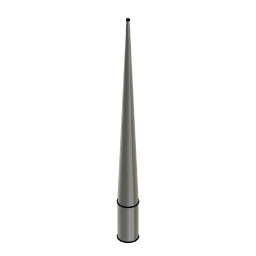
assembly_linear_actuator_no_spring (Autodesk Fusion 360 archive; units mm, degrees)
design "single tip press fit"
Autodesk Fusion 360 part; units mm, degrees
sketch "Sketch1" plane through (0, 0, 0) normal (0, 0, 1) x (1, 0, 0)
  circle A0 centre (0, 0) radius 1.5875
  dimension "d1" = 3.175
  dimension "d6" = 0
  constraint coincident A0.centre origin
  measures "d1" diameter of A0
ref_plane "WorkPlane1" through (0, 0, 33.02) normal (0, 0, 1) x (1, 0, 0)
sketch "Sketch2" plane through (0, 0, 33.02) normal (0, 0, 1) x (1, 0, 0)
  circle A0 centre (0, 0) radius 0.254
  dimension "d3" = 0.508
  constraint coincident A0.centre origin
  measures "d3" diameter of A0
loft "Loft1" add profiles "Sketch1", "Sketch2" section 1 section 2
extrude "Extrude2" add 1 faces at (-0.3879, 0.3599, 0) along direction (0, 0, -1) blind 6.35
sketch "Sketch4" plane through (0, 0, 0) normal (0, 1, 0) x (1, 0, 0)
equation "d1 = ( 1 / 8 ) * 1 in"

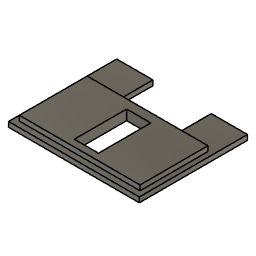
design "table_window"
Autodesk Fusion 360 part; units mm, degrees
sketch "Sketch1" plane through (0, 0, 0) normal (0, 0, 1) x (1, 0, 0)
  line L0 (0, 0) -> (76.2, 0)
  line L1 (76.2, 0) -> (76.2, 42.8752)
  line L2 (76.2, 42.8752) -> (0, 42.8752)
  line L3 (0, 42.8752) -> (0, 0)
  line L4 (38.1, 42.8752) -> (38.1, 0) construction
  line L5 (0, 21.4376) -> (76.2, 20.5486) construction
  line L6 (30.48, 4.2545) -> (45.72, 4.2545)
  line L7 (79.375, -3.6195) -> (-3.175, -3.6195)
  line L8 (-3.175, -3.6195) -> (-3.175, 45.6057)
  line L9 (-3.175, 45.6057) -> (79.375, 45.6057)
  line L10 (79.375, 45.6057) -> (79.375, -3.6195)
  line L11 (74.796, 42.8752) -> (79.375, 45.6057) construction
  line L12 (-3.175, -3.6195) -> (2.8949, 0) construction
  line L13 (79.375, -3.6195) -> (73.3051, 0) construction
  line L14 (1.404, 42.8752) -> (-3.175, 45.6057) construction
  line L15 (45.72, 37.2745) -> (30.48, 37.2745)
  line L16 (45.72, 37.2745) -> (45.72, 4.2545)
  line L17 (30.48, 37.2745) -> (30.48, 4.2545)
  dimension "d1" = 76.2
  dimension "d2" = 42.8752
  dimension "d3" = 15.24
  dimension "d5" = 82.55
  dimension "d6" = 49.2252
  constraint horizontal L0
  constraint vertical L1
  constraint horizontal L2
  constraint vertical L3
  constraint coincident L0.start L3.end
  constraint midpoint L2 L4.start
  constraint midpoint L0 L4.end
  constraint midpoint L3 L5.start
  constraint coincident L1 L5.end
  constraint horizontal L7
  constraint perpendicular L7 L8
  constraint parallel L7 L9
  constraint parallel L8 L10
  constraint coincident L2 L11.start
  constraint collinear L11 L12
  constraint coincident L0 L12.end
  constraint coincident L0 L13.end
  constraint collinear L13 L14
  constraint coincident L2 L14.start
  constraint horizontal L15
  constraint perpendicular L6 L17
  measures "d1" distance of L0.start L0.end
  measures "d2" distance of L0.start L2.end
  measures "d3" distance of L6.start L6.end
  measures "d5" distance of L8.end L9.end
  measures "d6" distance of L7.end L8.end
extrude "Extrude1" add sketch "Sketch1" along normal blind 6.35 contours L0 L1 L2 L3
extrude "Extrude2" add sketch "Sketch1" along normal blind 3.175 contours L7 L8 L9 L10
sketch "Sketch2" plane through (0, 45.6057, 0) normal (0, 1, 0) x (-1, 0, 0)
  line L0 (-79.375, 0) -> (3.175, 0)
  line L1 (3.175, 0) -> (3.175, 3.175)
  line L2 (3.175, 3.175) -> (-79.375, 3.175)
  line L3 (-79.375, 3.175) -> (-79.375, 0)
  line L4 (3.175, 0) -> (-19.685, 0)
  line L5 (-19.685, 0) -> (-19.685, 3.175)
  line L6 (-19.685, 3.175) -> (3.175, 3.175)
  line L7 (3.175, 3.175) -> (3.175, 0)
  line L8 (-79.375, 0) -> (-56.515, 0)
  line L9 (-56.515, 0) -> (-56.515, 3.175)
  line L10 (-56.515, 3.175) -> (-79.375, 3.175)
  line L11 (-79.375, 3.175) -> (-79.375, 0)
  dimension "d12" = 22.86
  dimension "d13" = 22.86
  constraint horizontal L4
  constraint vertical L5
  constraint horizontal L6
  constraint vertical L7
  constraint coincident L0.end L1.start
  constraint horizontal L8
  constraint vertical L9
  constraint horizontal L10
  constraint vertical L11
  constraint coincident L0.start L3.end
  measures "d12" distance of L0.end L4.end
  measures "d13" distance of L0.start L8.end
extrude "Extrude3" add sketch "Sketch2" along normal blind 19.05 contours L0 L2 L3 L8 L9 L10 L11 | L0 L1 L2 L4 L5 L6 L7

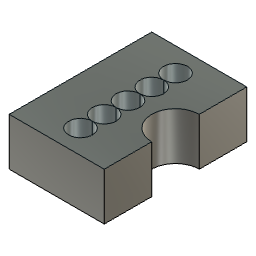
design "base for 5 tips press fit"
Autodesk Fusion 360 part; units mm, degrees
sketch "Sketch1" plane through (0, 0, 0) normal (0, 0, 1) x (1, 0, 0)
  line L0 (-6.35, 9.525) -> (6.35, 9.525)
  line L1 (6.35, 9.525) -> (6.35, -9.525)
  line L2 (6.35, -9.525) -> (-6.35, -9.525)
  line L3 (-6.35, -9.525) -> (-6.35, 9.525)
  line L4 (0, 0) -> (0, 3.175) construction
  line L5 (0, 3.175) -> (0, 6.35) construction
  line L6 (0, 0) -> (0, -3.175) construction
  line L7 (0, -3.175) -> (0, -6.35) construction
  circle A0 centre (0, 6.35) radius 1.5875
  circle A1 centre (0, 3.175) radius 1.5875
  circle A2 centre (0, 0) radius 1.5875
  circle A3 centre (0, -3.175) radius 1.5875
  circle A4 centre (0, -6.35) radius 1.5875
  arc A5 (6.35, 3.175) -> (6.35, -3.175) centre (6.35, 0) ccw
  dimension "d3" = 12.7
  dimension "d4" = 19.05
  dimension "d5" = 3.175
  dimension "d6" = 3.175
  dimension "d7" = 3.175
  dimension "d8" = 3.175
  dimension "d9" = 3.175
  dimension "d10" = 3.175
  dimension "d11" = 3.175
  dimension "d12" = 3.175
  dimension "d13" = 3.175
  dimension "d21" = 6.35
  constraint horizontal L0
  constraint vertical L1
  constraint horizontal L2
  constraint vertical L3
  constraint coincident L4.start L6.start
  constraint vertical L4
  constraint parallel L4 L5
  constraint parallel L4 L6
  constraint parallel L6 L7
  constraint coincident L5.end A0.centre
  constraint coincident L4.end L5.start
  constraint coincident L6.end L7.start
  constraint coincident L7.end A4.centre
  constraint midpoint L1 A5.centre
  constraint coincident L1 A5.end
  constraint coincident L1 A5.start
  measures "d3" distance of L0.start L0.end
  measures "d4" distance of L0.start L2.end
  measures "d5" distance of L4.start L4.end
  measures "d6" distance of L4.end L5.end
  measures "d7" distance of L4.start L6.end
  measures "d8" distance of L6.end L7.end
  measures "d9" diameter of A0
  measures "d10" diameter of A1
  measures "d11" diameter of A2
  measures "d12" diameter of A3
  measures "d13" diameter of A4
  measures "d21" diameter of A5
extrude "Extrude1" add sketch "Sketch1" along normal blind 6.35 contours L0 L1 L2 L3 A5
sketch "Sketch2" plane through (0, 0, 6.35) normal (0, 0, 1) x (-1, 0, 0)
  circle A0 centre (0, 6.35) radius 1.5875
  circle A1 centre (0, -6.35) radius 1.5875
  line L0 (6.35, 9.525) -> (-6.35, 9.525)
  line L1 (-6.35, -3.175) -> (-6.35, -9.525)
  line L2 (-6.35, -9.525) -> (6.35, -9.525)
  line L3 (6.35, -9.525) -> (6.35, 9.525)
  arc A2 (1.905, 6.35) -> (-1.905, 6.35) centre (0, 6.35) ccw
  arc A3 (-1.905, -6.35) -> (1.905, -6.35) centre (0, -6.35) ccw
  circle A4 centre (0, -3.175) radius 1.5875
  arc A5 (0, -1.5875) -> (0, 1.5875) centre (0, 0) ccw
  arc A6 (0, 1.5875) -> (0, 4.7625) centre (0, 3.175) ccw
  arc A7 (0, -1.5875) -> (0, -4.7625) centre (0, -3.175) ccw
  arc A8 (0, 1.5875) -> (0, -1.5875) centre (0, 0) ccw
  arc A9 (0, 4.7625) -> (0, 1.5875) centre (0, 3.175) ccw
  line L4 (-6.35, 9.525) -> (-6.35, 3.175)
  arc A10 (-6.35, -3.175) -> (-6.35, 3.175) centre (-6.35, 0) ccw
  dimension "d17" = 3.81
  dimension "d18" = 3.81
  constraint concentric A0 A2
  constraint coincident L3 A2.start
  constraint concentric A1 A3
  measures "d17" diameter of A2
  measures "d18" diameter of A3
sketch "Sketch3" plane through (0, 0, 6.35) normal (0, 0, 1) x (-1, 0, 0)
  circle A0 centre (0, 6.35) radius 1.5875
  arc A1 (0, 1.5875) -> (0, 4.7625) centre (0, 3.175) ccw
  arc A2 (0, -1.5875) -> (0, 1.5875) centre (0, 0) ccw
  arc A3 (0, -4.7625) -> (0, -1.5875) centre (0, -3.175) ccw
  circle A4 centre (0, -6.35) radius 1.5875
  arc A5 (0, -1.5875) -> (0, -4.7625) centre (0, -3.175) ccw
  arc A6 (0, 1.5875) -> (0, -1.5875) centre (0, 0) ccw
  arc A7 (0, 4.7625) -> (0, 1.5875) centre (0, 3.175) ccw
  line L0 (-6.35, -3.175) -> (-6.35, -9.525)
  line L1 (-6.35, -9.525) -> (6.35, -9.525)
  line L2 (6.35, -9.525) -> (6.35, 9.525)
  line L3 (6.35, 9.525) -> (-6.35, 9.525)
  line L4 (-6.35, 9.525) -> (-6.35, 3.175)
  arc A8 (-6.35, -3.175) -> (-6.35, 3.175) centre (-6.35, 0) ccw
sketch "Sketch4" plane through (-6.35, 0, 0) normal (-1, 0, 0) x (0, -1, 0)
  line L0 (-9.525, 0) -> (9.525, 0)
  line L1 (9.525, 0) -> (9.525, 6.35)
  line L2 (9.525, 6.35) -> (-9.525, 6.35)
  line L3 (-9.525, 6.35) -> (-9.525, 0)
  line L4 (0, 0) -> (0, 3.175) construction
  circle A0 centre (0, 3.175) radius 1.905
  dimension "d22" = 3.175
  dimension "d23" = 3.81
  constraint coincident L4.start origin
  constraint perpendicular L0 L4
  constraint coincident L4.end A0.centre
  measures "d22" distance of L4.start L4.end
  measures "d23" diameter of A0
extrude "Extrude3" cut sketch "Sketch4" against normal blind 3.81 contours A0
thread "Thread1" "ANSI Unified Screw Threads 0.164(#8) 8-32 UNC 3B" major diameter 4.1656 minor diameter 3.4163 pitch 0.7937 angle 60 resizes the face on face at (-3.81, -1.8955, 2.9853)
equation "d9 = ( 1 / 8 ) * 1 in"
equation "d10 = ( 1 / 8 ) * 1 in"
equation "d11 = ( 1 / 8 ) * 1 in"
equation "d13 = ( 1 / 8 ) * 1 in"
equation "d21 = ( 1 / 4 ) * 1 in"
equation "d22 = ( 1 / 8 ) * 1 in"

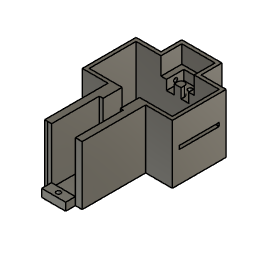
design "Circuit Base new"
Autodesk Fusion 360 part; units mm, degrees
sketch "Sketch1" plane through (0, 0, 0) normal (0, 0, 1) x (1, 0, 0)
  line L0 (76.2, 25.4) -> (0, 25.4)
  line L1 (48.6484, -35) -> (48.6484, -85)
  line L2 (26.6484, -76) -> (26.6484, -85)
  line L3 (48.6484, -76) -> (48.6484, -35)
  line L4 (26.6484, -35) -> (26.6484, -76)
  line L5 (30.1, -17.526) -> (30.1, -34.9936)
  line L6 (46.1, -34.9936) -> (46.1, -17.526)
  circle A0 centre (37.6484, -83.3194) radius 2.05
  line L7 (37.6484, -81.2694) -> (37.6484, -80.5) construction
  line L8 (48.6484, -76.0942) -> (48.6484, -35)
  line L9 (26.6484, -75.9063) -> (26.6484, -35)
  line L10 (46.1, -17.526) -> (46.1, -34.9936)
  line L11 (30.1, -34.9936) -> (26.6484, -34.9936)
  line L12 (30.1, -17.526) -> (30.1, -34.9936)
  line L13 (0, 25.4) -> (76.2, 25.4)
  line L14 (79.375, 28.575) -> (-3.175, 28.575)
  line L15 (30.1, -17.526) -> (30.1, -34.9936)
  line L16 (30.1, -34.9936) -> (26.6484, -34.9936)
  line L17 (26.6484, -34.9936) -> (26.6484, -75.9063)
  line L18 (46.1, -17.526) -> (46.1, -34.9936)
  line L19 (46.1, -34.9936) -> (48.6484, -34.9936)
  line L20 (48.6484, -34.9936) -> (48.6484, -76.0942)
  line L21 (46.1, -34.9936) -> (48.6484, -34.9936)
  line L22 (26.6484, -75.9063) -> (26.6484, -78.7257)
  line L23 (26.6484, -78.7257) -> (48.6484, -78.9136)
  line L24 (48.6484, -85) -> (48.6484, -78.9136)
  line L25 (48.6484, -76.0942) -> (48.6484, -76)
  line L26 (26.6484, -85) -> (26.6484, -78.7257)
  line L27 (26.6484, -75.9063) -> (26.6484, -35)
  line L28 (52.3234, -78.9136) -> (48.6484, -78.9136)
  line L29 (22.9734, -78.7257) -> (26.6484, -78.7257)
  line L30 (26.6484, -85) -> (26.6484, -87.8194)
  line L31 (48.6484, -85) -> (48.6484, -87.8194)
  line L32 (48.6484, -87.8194) -> (26.6484, -87.8194)
  line L33 (20.32, -78.74) -> (20.32, -66.04)
  line L34 (20.32, -66.04) -> (20.32, -20.701)
  line L35 (22.9734, -78.7257) -> (20.32, -78.74)
  line L36 (52.3234, -78.9136) -> (54.8634, -78.9136)
  line L37 (54.8634, -78.9136) -> (54.8634, -20.701)
  line L38 (-3.1761, -11.938) -> (-3.175, -11.938)
  line L39 (76.1981, -17.526) -> (46.1, -17.526)
  line L40 (30.1, -17.526) -> (0, -17.526)
  line L41 (-3.173, -20.701) -> (20.32, -20.701)
  line L42 (54.8634, -20.701) -> (79.3731, -20.701)
  line L43 (76.2, 25.4) -> (76.1981, -17.526)
  line L44 (79.375, 28.575) -> (79.3731, -20.701)
  line L45 (0, 25.4) -> (0, -17.526)
  line L46 (-3.175, 28.575) -> (-3.173, -20.701)
  point P0 (38.1, 0)
  point P1 (38.1, -15)
  point P2 (37.6484, 0)
  dimension "d2" = 25.4
  dimension "d5" = 9
  dimension "d6" = 41
  dimension "d9" = 16
  dimension "d12" = 4.1
  dimension "d47" = 2.8194
  dimension "d48" = 2.8194
  dimension "d50" = 2.8194
  dimension "d51" = 2.8194
  dimension "d53" = 2.54
  constraint horizontal L0
  constraint vertical L1
  constraint vertical L26
  constraint vertical L24
  constraint vertical L2
  constraint vertical L3
  constraint vertical L4
  constraint parallel L5 L6
  constraint vertical L8
  constraint vertical L9
  constraint horizontal L21
  constraint vertical L10
  constraint horizontal L11
  constraint vertical L12
  constraint horizontal L13
  constraint horizontal L14
  constraint vertical L15
  constraint horizontal L16
  constraint vertical L17
  constraint vertical L18
  constraint horizontal L19
  constraint vertical L20
  constraint collinear L24 L25
  constraint collinear L26 L27
  constraint coincident A0 L7.start
  constraint perpendicular L29 L33
  constraint coincident L5.start L39
  constraint collinear L39 L40
  constraint collinear L41 L42
  constraint vertical L45
  measures "d2" distance of origin L0.end
  measures "d5" distance of L2.end L2.start
  measures "d6" distance of L2.start L4.start
  measures "d9" distance of L5.end L6.start
  measures "d12" diameter of A0
  measures "d47" distance of L9.start L22.end
  measures "d48" distance of L8.start L23.end
  measures "d50" distance of L2.end L30.end
  measures "d51" distance of L1.end L31.end
  measures "d53" distance of L28.start L36.end
extrude "Extrude7" add sketch "Sketch1" against normal blind 3.175 makes body 1
extrude "Extrude8" add sketch "Sketch1" along normal blind 50.8 contours L0 L1 L2 L3 L4 L5 L6 L8 L9 L10 L11 L12 L13 L14 L15 L16 L17 L18 L19 L20 L21 L22 L25 L27 L28 L29 L33 L34 L35 L36 L37 L39 L40 L41 L42 L43 L44 L45 L46 bodies 1
extrude "Extrude10" add sketch "Sketch1" along normal blind 4 contours L1 L2 L23 L24 L26 L30 L31 L32 bodies 1
sketch "Sketch3" plane through (0, 28.575, 0) normal (0, 1, 0) x (-1, 0, 0)
  line L0 (-79.375, 50.8) -> (-79.375, -3.175)
  line L1 (-79.375, -3.175) -> (3.175, -3.175)
  line L2 (3.175, -3.175) -> (3.175, 50.8)
  line L3 (3.175, 50.8) -> (-79.375, 50.8)
  line L4 (-53.34, 20.32) -> (-22.86, 20.32)
  line L5 (-22.86, 20.32) -> (-22.86, 34.6202)
  line L6 (-22.86, 34.6202) -> (-53.34, 34.6202)
  line L7 (-53.34, 34.6202) -> (-53.34, 20.32)
  dimension "d87" = 30.48
  dimension "d88" = 14.3002
  constraint horizontal L4
  constraint vertical L5
  constraint horizontal L6
  constraint vertical L7
  measures "d87" distance of L4.start L4.end
  measures "d88" distance of L4.start L6.end
extrude "Extrude11" add sketch "Sketch3" along normal blind 15.875 separate body contours L4 L5 L6 L7 makes body 2
sketch "Sketch4" plane through (0, 0, 34.6202) normal (0, 0, 1) x (-1, 0, 0)
  line L0 (-22.86, -28.575) -> (-53.34, -28.575)
  line L1 (-53.34, -28.575) -> (-53.34, -44.45)
  line L2 (-53.34, -44.45) -> (-22.86, -44.45)
  line L3 (-22.86, -44.45) -> (-22.86, -28.575)
  line L4 (-48.26, -28.575) -> (-27.94, -28.575)
  line L5 (-27.94, -28.575) -> (-27.94, -41.275)
  line L6 (-27.94, -41.275) -> (-48.26, -41.275)
  line L7 (-48.26, -41.275) -> (-48.26, -28.575)
  circle A0 centre (-38.1, -28.575) radius 3.175
  dimension "d91" = 20.32
  dimension "d92" = 12.7
  dimension "d93" = 5.08
  dimension "d94" = 6.35
  constraint horizontal L4
  constraint vertical L5
  constraint horizontal L6
  constraint vertical L7
  constraint coincident L0 L4.start
  constraint midpoint L4 A0.centre
  measures "d91" distance of L4.start L4.end
  measures "d92" distance of L4.start L6.end
  measures "d93" distance of L3 L5
  measures "d94" diameter of A0
extrude "Extrude12" cut sketch "Sketch4" against normal blind 8.89 contours L0 L4 L5 L6 L7 A0 bodies 2
sketch "Sketch5" plane through (22.86, 0, 0) normal (-1, 0, 0) x (0, -1, 0)
  line L0 (-28.575, 20.32) -> (-28.575, 34.6202)
  line L1 (-28.575, 34.6202) -> (-44.45, 34.6202)
  line L2 (-44.45, 34.6202) -> (-44.45, 20.32)
  line L3 (-44.45, 20.32) -> (-28.575, 20.32)
  circle A0 centre (-33.7311, 29.984) radius 1.778
  dimension "d97" = 3.556
  measures "d97" diameter of A0
extrude "Extrude13" cut sketch "Sketch5" against normal blind 48.26 contours A0 bodies 2
extrude "Extrude14" add 1 faces at (43.18, 44.45, 25.0867) along direction (0, 1, 0) blind 3.175 on bodies 2 bodies 2
extrude "Extrude15" add 1 faces at (22.86, 43.56, 28.1334) along direction (-1, 0, 0) blind 3.175 on bodies 2 bodies 1 2
extrude "Extrude16" add 1 faces at (53.34, 43.56, 28.1334) along direction (1, 0, 0) blind 3.175 on bodies 1 bodies 1
extrude "Extrude17" add 1 faces at (22.4367, 39.1583, 34.6202) along direction (0, 0, 1) up to surface (16.1798 mm away) on bodies 1 bodies 1
sketch "Sketch6" plane through (0, 0, 50.8) normal (0, 0, 1) x (-1, 0, 0)
  line L0 (-48.26, -28.575) -> (-27.94, -28.575)
  line L1 (-27.94, -28.575) -> (-27.94, -41.275)
  line L2 (-27.94, -41.275) -> (-48.26, -41.275)
  line L3 (-48.26, -41.275) -> (-48.26, -28.575)
  line L4 (-56.515, -28.575) -> (-56.515, -47.625)
  line L5 (-56.515, -47.625) -> (-19.685, -47.625)
  line L6 (-19.685, -47.625) -> (-19.685, -28.575)
  line L7 (-19.685, -28.575) -> (3.175, -28.575)
  line L8 (3.175, -28.575) -> (3.173, 20.701)
  line L9 (3.173, 20.701) -> (-20.32, 20.701)
  line L10 (-20.32, 20.701) -> (-20.32, 78.74)
  line L11 (-20.32, 78.74) -> (-22.9734, 78.7257)
  line L12 (-22.9734, 78.7257) -> (-26.6484, 78.7257)
  line L13 (-26.6484, 78.7257) -> (-26.6484, 34.9936)
  line L14 (-26.6484, 34.9936) -> (-30.1, 34.9936)
  line L15 (-30.1, 34.9936) -> (-30.1, 17.526)
  line L16 (-30.1, 17.526) -> (0, 17.526)
  line L17 (0, 17.526) -> (0, -25.4)
  line L18 (0, -25.4) -> (-76.2, -25.4)
  line L19 (-76.2, -25.4) -> (-76.1981, 17.526)
  line L20 (-76.1981, 17.526) -> (-46.1, 17.526)
  line L21 (-46.1, 17.526) -> (-46.1, 34.9936)
  line L22 (-46.1, 34.9936) -> (-48.6484, 34.9936)
  line L23 (-48.6484, 34.9936) -> (-48.6484, 78.9136)
  line L24 (-48.6484, 78.9136) -> (-54.8634, 78.9136)
  line L25 (-54.8634, 78.9136) -> (-54.8634, 20.701)
  line L26 (-54.8634, 20.701) -> (-79.3731, 20.701)
  line L27 (-79.3731, 20.701) -> (-79.375, -28.575)
  line L28 (-79.375, -28.575) -> (-56.515, -28.575)
  line L29 (-53.34, -28.575) -> (-22.86, -28.575)
  line L30 (-22.86, -28.575) -> (-22.86, -44.45)
  line L31 (-22.86, -44.45) -> (-53.34, -44.45)
  line L32 (-53.34, -44.45) -> (-53.34, -28.575)
  dimension "d108" = 30.48
  dimension "d109" = 15.875
  dimension "d110" = 3.175
  dimension "d111" = 3.175
  constraint horizontal L29
  constraint vertical L30
  constraint horizontal L31
  constraint vertical L32
  measures "d108" distance of L29.start L29.end
  measures "d109" distance of L29.start L31.end
  measures "d110" distance of L4 L32
  measures "d111" distance of L5 L31
extrude "Extrude18" cut sketch "Sketch6" against normal up to surface (16.1798 mm away) contours L1 L2 L3 L29 L30 L31 L32 bodies 1
extrude "Extrude19" add 1 faces at (44.2383, 34.925, 20.32) along direction (0, 0, -1) up to surface (23.495 mm away) thin wall 3.175 inside on bodies 1 bodies 1
extrude "Extrude20" cut 1 faces at (37.0417, 28.575, 45.4067) along direction (0, -1, 0) blind 10.16 on bodies 1 bodies 1
sketch "Sketch7" plane through (0, 0, 25.7302) normal (0, 0, 1) x (-1, 0, 0)
  arc A0 (-41.275, -28.575) -> (-34.925, -28.575) centre (-38.1, -28.575) ccw
  line L0 (-41.275, -28.575) -> (-41.275, -25.4)
  line L1 (-41.275, -25.4) -> (-48.26, -25.4)
  line L2 (-27.94, -25.4) -> (-34.925, -25.4)
  line L3 (-34.925, -25.4) -> (-34.925, -28.575)
  circle A1 centre (-38.1, -36.9824) radius 2.0447
  line L4 (-48.26, -25.4) -> (-48.26, -41.275)
  line L5 (-48.26, -41.275) -> (-27.94, -41.275)
  line L6 (-27.94, -41.275) -> (-27.94, -25.4)
  line L7 (-22.86, -44.45) -> (-53.34, -44.45)
  dimension "d119" = 4.0894
  dimension "d121" = 7.4676
  measures "d119" diameter of A1
  measures "d121" distance of A1.centre L7
extrude "Extrude21" cut sketch "Sketch7" against normal blind 15.24 contours A1 bodies 1
sketch "Sketch8" plane through (79.3739, -0.0031, 0) normal (1, -0.000039, 0) x (0.000039, 1, 0)
  line L0 (-20.6979, 50.8) -> (-20.6979, -3.175)
  line L1 (-20.6979, -3.175) -> (28.5781, -3.175)
  line L2 (28.5781, -3.175) -> (28.5781, 50.8)
  line L3 (28.5781, 50.8) -> (-20.6979, 50.8)
  line L4 (-14.3479, 27.686) -> (22.2281, 27.686)
  line L5 (22.2281, 27.686) -> (22.2281, 24.511)
  line L6 (22.2281, 24.511) -> (-14.3479, 24.511)
  line L7 (-14.3479, 24.511) -> (-14.3479, 27.686)
  dimension "d124" = 27.686
  dimension "d125" = 6.35
  dimension "d126" = 6.35
  dimension "d129" = 3.175
  constraint horizontal L4
  constraint vertical L5
  constraint horizontal L6
  constraint vertical L7
  measures "d124" distance of L1 L6
  measures "d125" distance of L2 L5
  measures "d126" distance of L0 L7
  measures "d129" distance of L4.start L6.end
extrude "Extrude22" cut sketch "Sketch8" along normal mid plane 22.86 contours L4 L5 L6 L7 bodies 1
sketch "Sketch2" plane through (0, 0, 0) normal (0, 0, 1) x (1, 0, 0)
  line L0 (0, 25.4) -> (76.2, 25.4)
  line L1 (76.2, 25.4) -> (76.2, -11.938)
  line L2 (76.2, -11.938) -> (0, -11.938)
  line L3 (0, -11.938) -> (0, 25.4)
  line L4 (0, 25.4) -> (76.2, 25.4)
  line L5 (76.2, 25.4) -> (76.2, -11.938)
  line L6 (76.2, -11.938) -> (0, -11.938)
  line L7 (0, -11.938) -> (0, 25.4)
  line L8 (-3.175, 28.575) -> (79.375, 28.575)
  line L9 (79.375, 28.575) -> (79.375, -15.113)
  line L10 (-3.175, -15.113) -> (-3.175, 28.575)
  line L11 (-3.175, -15.113) -> (-3.175, -20.701)
  line L12 (79.375, -15.113) -> (79.375, -20.701)
  line L13 (79.375, -20.701) -> (-3.175, -20.701)
  line L14 (0, -11.938) -> (0, -17.526)
  line L15 (76.2, -11.938) -> (76.2, -17.526)
  line L16 (76.2, -17.526) -> (0, -17.526)
  line L17 (79.375, -15.113) -> (76.2, -15.113)
  line L18 (0, -15.113) -> (-3.175, -15.113)
  dimension "d67" = 82.55
  dimension "d68" = 43.688
  dimension "d69" = 3.175
  dimension "d70" = 3.175
  dimension "d71" = 5.588
  dimension "d72" = 5.588
  dimension "d73" = 5.588
  dimension "d74" = 5.588
  constraint horizontal L0
  constraint vertical L1
  constraint horizontal L2
  constraint vertical L3
  constraint horizontal L4
  constraint vertical L5
  constraint horizontal L6
  constraint vertical L7
  constraint horizontal L8
  constraint vertical L9
  constraint horizontal L17
  constraint vertical L10
  constraint perpendicular L11 L17
  constraint perpendicular L12 L17
  constraint perpendicular L14 L17
  constraint perpendicular L15 L17
  constraint coincident L15 L17.end
  constraint coincident L14 L18.start
  constraint collinear L17 L18
  measures "d67" distance of L8.start L8.end
  measures "d68" distance of L8.start L10.start
  measures "d69" distance of L0 L8
  measures "d70" distance of L3 L10
  measures "d71" distance of L10.start L11.end
  measures "d72" distance of L9.end L12.end
  measures "d73" distance of L2.end L14.end
  measures "d74" distance of L1.end L15.end
extrude "Extrude1" [suppressed]
extrude "Extrude9" [suppressed]
extrude "Extrude2" [suppressed]
extrude "Extrude4" [suppressed]
extrude "Extrude5" [suppressed]
extrude "Extrude6" [suppressed]
extrude "Extrude3" [suppressed]

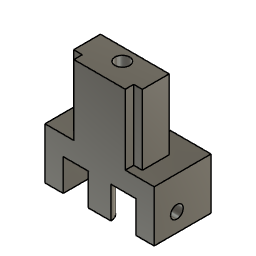
design "tip_holder_puzzle"
Autodesk Fusion 360 part; units mm, degrees
sketch "Sketch1" plane through (0, 0, 0) normal (0, 0, 1) x (1, 0, 0)
  line L0 (0, 0) -> (26.67, 0)
  line L1 (26.67, 0) -> (26.67, 12.7)
  line L2 (26.67, 12.7) -> (0, 12.7)
  line L3 (0, 12.7) -> (0, 0)
  line L4 (0, 0) -> (3.175, 0)
  line L5 (3.175, 0) -> (3.175, 12.7)
  line L6 (3.175, 12.7) -> (0, 12.7)
  line L7 (0, 12.7) -> (0, 0)
  line L8 (26.67, 0) -> (23.495, 0)
  line L9 (23.495, 0) -> (23.495, 12.7)
  line L10 (23.495, 12.7) -> (26.67, 12.7)
  line L11 (26.67, 12.7) -> (26.67, 0)
  circle A0 centre (13.335, 6.35) radius 2.05
  line L12 (13.335, 12.7) -> (13.335, 0) construction
  line L13 (3.175, 6.35) -> (23.495, 6.35) construction
  point P0 (13.335, 6.35)
  dimension "d1" = 26.67
  dimension "d2" = 12.7
  dimension "d3" = 3.175
  dimension "d4" = 3.175
  dimension "d5" = 4.1
  constraint horizontal L0
  constraint vertical L1
  constraint horizontal L2
  constraint vertical L3
  constraint coincident L0.start L3.end
  constraint horizontal L4
  constraint vertical L5
  constraint horizontal L6
  constraint vertical L7
  constraint horizontal L8
  constraint vertical L9
  constraint horizontal L10
  constraint vertical L11
  constraint midpoint L2 L12.start
  constraint midpoint L0 L12.end
  constraint midpoint L5 L13.start
  constraint midpoint L9 L13.end
  constraint midpoint L13 P0
  measures "d1" distance of L0.start L0.end
  measures "d2" distance of L0.start L2.end
  measures "d3" distance of L0.start L4.end
  measures "d4" distance of L0.end L8.end
  measures "d5" diameter of A0
extrude "Extrude1" add sketch "Sketch1" along normal blind 5.4
extrude "Extrude3" add sketch "Sketch1" against normal blind 7.62 contours L0 L1 L2 L8 L9 L10 L11
extrude "Extrude4" add sketch "Sketch1" against normal blind 8.89 contours L0 L2 L3 L4 L5 L6 L7
ref_plane "WorkPlane1" through (13.335, 6.35, 2.21) normal (0, 0, 1) x (1, 0, 0)
sketch "Sketch2" plane through (0, 0, 2.21) normal (0, 0, 1) x (1, 0, 0)
  circle A0 centre (13.3518, 6.366) radius 2.05
  dimension "d15" = 4.1
  measures "d15" diameter of A0
sketch "Sketch3" plane through (0, 0, 0) normal (0, 0, 1) x (1, 0, 0)
  circle A0 centre (13.335, 6.35) radius 4
  circle A1 centre (13.335, 6.35) radius 2.05
  dimension "d16" = 8
  constraint concentric A0 A1
  measures "d16" diameter of A0
loft "Loft1" cut profiles "Sketch3", "Sketch2" section 1 section 2
sketch "Sketch4" plane through (23.495, 0, 0) normal (-1, 0, 0) x (0, -1, 0)
  line L0 (0, 0) -> (-12.7, 0)
  line L1 (-12.7, 0) -> (-12.7, -7.62)
  line L2 (-12.7, -7.62) -> (0, -7.62)
  line L3 (0, -7.62) -> (0, 0)
  circle A0 centre (-6.35, -3.81) radius 1.778
  dimension "d17" = 3.556
  measures "d17" diameter of A0
extrude "Extrude5" cut sketch "Sketch4" along normal blind 26 and the other way blind 17 contours A0
sketch "Sketch5" plane through (0, 0, 5.4) normal (0, 0, 1) x (-1, 0, 0)
  circle A0 centre (-13.335, -6.35) radius 2.05
  line L0 (-26.67, -12.7) -> (0, -12.7)
  line L1 (0, -12.7) -> (0, 0)
  line L2 (0, 0) -> (-26.67, 0)
  line L3 (-26.67, 0) -> (-26.67, -12.7)
  line L4 (-13.335, 0) -> (-13.335, -12.7) construction
  line L5 (0, -6.35) -> (-26.67, -6.35) construction
  line L6 (-6.1595, -2.3495) -> (-20.5105, -2.3495)
  line L7 (-20.5105, -2.3495) -> (-20.5105, -10.3505)
  line L8 (-20.5105, -10.3505) -> (-6.1595, -10.3505)
  line L9 (-6.1595, -10.3505) -> (-6.1595, -2.3495)
  line L10 (-6.1595, -2.3495) -> (-20.5105, -10.3505) construction
  line L11 (-20.5105, -2.3495) -> (-6.1595, -10.3505) construction
  line L12 (-20.5105, -2.3495) -> (-6.1595, -2.3495)
  point P0 (-13.335, -6.35)
  point P1 (-13.335, -6.35)
  dimension "d26" = 14.351
  dimension "d27" = 8.001
  dimension "d28" = 14.351
  constraint midpoint L2 L4.start
  constraint midpoint L0 L4.end
  constraint midpoint L1 L5.start
  constraint midpoint L3 L5.end
  constraint coincident P0 A0.centre
  constraint horizontal L6
  constraint perpendicular L6 L7
  constraint parallel L6 L8
  constraint parallel L7 L9
  constraint coincident L10 P1
  constraint coincident L11 P1
  constraint horizontal L12
  measures "d26" distance of L7.end L8.end
  measures "d27" distance of L6.end L7.end
  measures "d28" distance of L6.end L6.start
extrude "Extrude6" add sketch "Sketch5" along normal blind 8.128 contours L6 L7 L8 L9 L12
sketch "Sketch6" plane through (0, 0, 13.528) normal (0, 0, 1) x (-1, 0, 0)
  circle A0 centre (-13.335, -6.35) radius 2.05
  line L0 (-6.1595, -2.3495) -> (-20.5105, -2.3495)
  line L1 (-20.5105, -2.3495) -> (-20.5105, -10.3505)
  line L2 (-20.5105, -10.3505) -> (-6.1595, -10.3505)
  line L3 (-6.1595, -10.3505) -> (-6.1595, -2.3495)
  line L4 (-20.5105, -2.3495) -> (-6.1595, -2.3495)
  line L5 (-6.1595, -2.3495) -> (-6.1595, 0.9525)
  line L6 (-6.1595, 0.9525) -> (-20.5105, 0.9525)
  line L7 (-20.5105, 0.9525) -> (-20.5105, -2.3495)
  line L8 (-3.7465, -2.3495) -> (-22.9235, -2.3495)
  line L9 (-22.9235, -2.3495) -> (-22.9235, -10.3505)
  line L10 (-22.9235, -10.3505) -> (-3.7465, -10.3505)
  line L11 (-3.7465, -10.3505) -> (-3.7465, -2.3495)
  line L12 (-3.7465, -2.3495) -> (-22.9235, -10.3505) construction
  line L13 (-22.9235, -2.3495) -> (-3.7465, -10.3505) construction
  point P0 (-13.335, -6.35)
  dimension "d30" = 14.351
  dimension "d31" = 3.302
  dimension "d32" = 19.177
  dimension "d33" = 8.001
  constraint horizontal L4
  constraint vertical L5
  constraint horizontal L6
  constraint vertical L7
  constraint coincident L0.end L1.start
  constraint horizontal L8
  constraint perpendicular L8 L9
  constraint parallel L8 L10
  constraint parallel L9 L11
  constraint coincident L12 P0
  constraint coincident L13 P0
  constraint coincident P0 A0.centre
  measures "d30" distance of L0.end L0.start
  measures "d31" distance of L0.end L6.end
  measures "d32" distance of L9.end L10.end
  measures "d33" distance of L8.end L9.end
extrude "Extrude7" add sketch "Sketch6" along normal blind -3.175 and the other way blind -11.43
sketch "Sketch7" plane through (0, 0, 24.958) normal (0, 0, 1) x (-1, 0, 0)
  circle A0 centre (-13.335, -6.35) radius 2.05
  line L0 (-22.9235, -10.3505) -> (-3.7465, -10.3505)
  line L1 (-3.7465, -10.3505) -> (-3.7465, -2.3495)
  line L2 (-3.7465, -2.3495) -> (-6.1595, -2.3495)
  line L3 (-6.1595, -2.3495) -> (-6.1595, 0.9525)
  line L4 (-6.1595, 0.9525) -> (-20.5105, 0.9525)
  line L5 (-20.5105, 0.9525) -> (-20.5105, -2.3495)
  line L6 (-20.5105, -2.3495) -> (-22.9235, -2.3495)
  line L7 (-22.9235, -2.3495) -> (-22.9235, -10.3505)
  line L8 (-13.335, -6.35) -> (-7.5565, -6.35) construction
  line L9 (-13.335, -6.35) -> (-9.3345, -6.35) construction
  line L10 (-17.3355, -2.3495) -> (-9.3345, -2.3495)
  line L11 (-9.3345, -6.35) -> (-9.3345, -2.3495) construction
  line L12 (-9.3345, -6.35) -> (-9.3345, -10.3505) construction
  arc A1 (-9.3345, -10.3505) -> (-9.3345, -2.3495) centre (-12.9461, -6.35) ccw
  line L13 (-13.335, -6.35) -> (-19.1135, -6.35) construction
  line L14 (-13.335, -6.35) -> (-17.3355, -6.35) construction
  line L15 (-17.3355, -6.35) -> (-17.3355, -2.3495) construction
  line L16 (-17.3355, -6.35) -> (-17.3355, -10.3505) construction
  arc A2 (-17.3355, -2.3495) -> (-17.3355, -10.3505) centre (-13.7239, -6.35) ccw
  dimension "d36" = 5.7785
  dimension "d37" = 4.0005
  dimension "d38" = 5.7785
  dimension "d39" = 4.0005
  constraint coincident A0.centre L8.start
  constraint horizontal L8
  constraint parallel L8 L9
  constraint perpendicular L10 L11
  constraint coincident L0 L12.end
  constraint perpendicular L0 L12
  constraint coincident L8.end A1
  constraint parallel L8 L13
  constraint parallel L13 L14
  constraint perpendicular L10 L15
  constraint coincident L0 L16.end
  constraint perpendicular L0 L16
  constraint coincident L13.end A2
  measures "d36" distance of A0.centre L8.end
  measures "d37" distance of A0.centre L9.end
  measures "d38" distance of A0.centre L13.end
  measures "d39" distance of A0.centre L14.end
sketch "Sketch9" plane through (0, 10.3505, 0) normal (0, 1, 0) x (-1, 0, 0)
  line L0 (-20.5105, 10.353) -> (-20.5105, 5.4)
  line L1 (-20.5105, 5.4) -> (-6.1595, 5.4)
  line L2 (-6.1595, 5.4) -> (-6.1595, 10.353)
  line L3 (-6.1595, 10.353) -> (-3.7465, 10.353)
  line L4 (-3.7465, 10.353) -> (-3.7465, 24.958)
  line L5 (-3.7465, 24.958) -> (-22.9235, 24.958)
  line L6 (-22.9235, 24.958) -> (-22.9235, 10.353)
  line L7 (-22.9235, 10.353) -> (-20.5105, 10.353)
  line L8 (-17.3355, 14.4805) -> (-9.3345, 14.4805)
  line L9 (-9.3345, 20.8305) -> (-17.3355, 20.8305)
  arc A0 (-9.3345, 14.4805) -> (-9.3345, 20.8305) centre (-19.0024, 17.6555) ccw
  arc A1 (-17.3355, 20.8305) -> (-17.3355, 14.4805) centre (-7.6676, 17.6555) ccw
  line L10 (-17.8435, 15.494) -> (-17.6113, 15.494) construction
  line L11 (-13.335, 24.958) -> (-13.335, 20.8305) construction
  line L12 (-13.335, 14.4805) -> (-13.335, 10.16) construction
  line L13 (-22.9235, 17.6555) -> (-17.8435, 17.6555) construction
  line L14 (-8.8265, 17.6555) -> (-3.7465, 17.6555) construction
  line L15 (-20.5105, 10.353) -> (-20.5105, 5.4)
  line L16 (-20.5105, 5.4) -> (-6.1595, 5.4)
  line L17 (-6.1595, 5.4) -> (-6.1595, 10.353)
  line L18 (-6.1595, 10.353) -> (-3.7465, 10.353)
  line L19 (-3.7465, 10.353) -> (-3.7465, 24.958)
  line L20 (-3.7465, 24.958) -> (-22.9235, 24.958)
  line L21 (-22.9235, 24.958) -> (-22.9235, 10.353)
  line L22 (-22.9235, 10.353) -> (-20.5105, 10.353)
  line L23 (-6.1595, 24.958) -> (-6.1595, 10.353)
  line L24 (-6.1595, 10.353) -> (-20.5105, 10.353)
  line L25 (-20.5105, 10.353) -> (-20.5105, 24.958)
  line L26 (-20.5105, 24.958) -> (-6.1595, 24.958)
  line L27 (-20.5105, 10.353) -> (-20.5105, 5.4)
  line L28 (-20.5105, 5.4) -> (-6.1595, 5.4)
  line L29 (-6.1595, 5.4) -> (-6.1595, 10.353)
  line L30 (-6.1595, 10.353) -> (-3.7465, 10.353)
  line L31 (-3.7465, 10.353) -> (-3.7465, 24.958)
  line L32 (-3.7465, 24.958) -> (-22.9235, 24.958)
  line L33 (-22.9235, 24.958) -> (-22.9235, 10.353)
  line L34 (-22.9235, 10.353) -> (-20.5105, 10.353)
  point P0 (-13.335, 17.6555)
  dimension "d56" = 8.001
  dimension "d57" = 6.35
  constraint midpoint L6 L13.start
  constraint midpoint L4 L14.end
  constraint midpoint L5 L11.start
  constraint perpendicular L11 L13
  constraint horizontal L8
  constraint parallel L8 L9
  constraint horizontal L10
  constraint coincident A1 L10.end
  constraint collinear L11 L12
  constraint coincident L8 L12.start
  constraint coincident A1 L13.end
  constraint coincident A0 L14.start
  constraint collinear L13 L14
  constraint coincident L9 L11.end
  measures "d56" distance of L9.start L9.end
  measures "d57" distance of L8.end L9.start
extrude "Extrude11" cut sketch "Sketch9" against normal blind 8.001 contours L8 L9 A0 A1
extrude "Extrude12" add 3 faces at (10.9432, 1.2488, 10.353) (4.5508, 7.6835, 10.353) (21.3148, 7.6835, 10.353) along direction (0, 0, -1) blind 4.953
extrude "Extrude13" add 1 faces at (26.67, 6.3943, 2.921) along direction (1, 0, 0) blind 1.905
extrude "Extrude14" add 1 faces at (0, 6.3057, 2.921) along direction (-1, 0, 0) blind 1.905
sketch "Sketch10" plane through (0, 0, 0) normal (0, 0, -1) x (1, 0, 0)
  circle A0 centre (13.335, -6.35) radius 4
  line L0 (3.175, 0) -> (3.175, -12.7)
  line L1 (3.175, -12.7) -> (23.495, -12.7)
  line L2 (23.495, -12.7) -> (23.495, 0)
  line L3 (23.495, 0) -> (3.175, 0)
  circle A1 centre (13.335, 0) radius 3.175
  dimension "d69" = 6.35
  constraint midpoint L3 A1.centre
  measures "d69" diameter of A1
extrude "Extrude15" cut 1 faces at (10.9432, -0.3175, 5.4) along direction (0, 0, 1) blind 26.67
extrude "Extrude16" add sketch "Sketch10" along normal up to surface (8.89 mm away) contours A0 A1 | A0 L3 A1 picked at (13.6688, -2.6285)
extrude "Extrude17" add 1 faces at (16.7217, 12.7, 3.6) along direction (0, 1, 0) blind 3.175
sketch "Sketch11" plane through (0, 0, 0) normal (0, 0, -1) x (1, 0, 0)
  arc A0 (14.991, -2.7089) -> (16.51, 0) centre (13.335, 0) ccw
  arc A1 (11.679, -2.7089) -> (14.991, -2.7089) centre (13.335, -6.35) ccw
  arc A2 (10.16, 0) -> (11.679, -2.7089) centre (13.335, 0) ccw
  line L0 (10.16, 0) -> (3.175, 0)
  line L1 (3.175, 0) -> (3.175, -15.875)
  line L2 (3.175, -15.875) -> (23.495, -15.875)
  line L3 (23.495, -15.875) -> (23.495, 0)
  line L4 (23.495, 0) -> (16.51, 0)
  line L5 (3.175, -15.875) -> (8.255, -15.875)
  line L6 (8.255, -15.875) -> (8.255, -12.7)
  line L7 (8.255, -12.7) -> (3.175, -12.7)
  line L8 (3.175, -12.7) -> (3.175, -15.875)
  line L9 (23.495, -15.875) -> (18.415, -15.875)
  line L10 (18.415, -15.875) -> (18.415, -12.7)
  line L11 (18.415, -12.7) -> (23.495, -12.7)
  line L12 (23.495, -12.7) -> (23.495, -15.875)
  dimension "d74" = 5.08
  dimension "d75" = 3.175
  dimension "d76" = 5.08
  dimension "d77" = 3.175
  constraint horizontal L5
  constraint vertical L6
  constraint horizontal L7
  constraint vertical L8
  constraint coincident L1.end L2.start
  constraint horizontal L9
  constraint vertical L10
  constraint horizontal L11
  constraint vertical L12
  constraint coincident L2.end L3.start
  measures "d74" distance of L1.end L5.end
  measures "d75" distance of L1.end L7.end
  measures "d76" distance of L2.end L9.end
  measures "d77" distance of L2.end L11.end
extrude "Extrude18" add sketch "Sketch11" along normal up to surface (8.89 mm away) contours L2 L3 L9 L10 L11 L12 | L1 L2 L5 L6 L7 L8
sketch "Sketch12" plane through (0, 0, 0) normal (0, 0, -1) x (1, 0, 0)
  line L0 (3.175, -12.7) -> (8.255, -12.7)
  line L1 (8.255, -12.7) -> (8.255, -15.875)
  line L2 (8.255, -15.875) -> (18.415, -15.875)
  line L3 (18.415, -15.875) -> (18.415, -12.7)
  line L4 (18.415, -12.7) -> (23.495, -12.7)
  line L5 (23.495, -12.7) -> (23.495, 0)
  line L6 (23.495, 0) -> (16.51, 0)
  arc A0 (14.991, -2.7089) -> (16.51, 0) centre (13.335, 0) ccw
  arc A1 (11.679, -2.7089) -> (14.991, -2.7089) centre (13.335, -6.35) ccw
  arc A2 (10.16, 0) -> (11.679, -2.7089) centre (13.335, 0) ccw
  line L7 (10.16, 0) -> (3.175, 0)
  line L8 (3.175, 0) -> (3.175, -12.7)
  circle A3 centre (13.335, -6.35) radius 4
  constraint concentric A1 A3
extrude "Extrude19" cut sketch "Sketch12" along normal blind 20.32 contours A1 A3
sketch "Sketch13" plane through (0, 0, 24.958) normal (0, 0, 1) x (-1, 0, 0)
  line L0 (-6.1595, 0) -> (-20.5105, 0)
  line L1 (-20.5105, 0) -> (-20.5105, -2.3495)
  line L2 (-20.5105, -2.3495) -> (-22.9235, -2.3495)
  line L3 (-22.9235, -2.3495) -> (-22.9235, -10.3505)
  line L4 (-22.9235, -10.3505) -> (-3.7465, -10.3505)
  line L5 (-3.7465, -10.3505) -> (-3.7465, -2.3495)
  line L6 (-3.7465, -2.3495) -> (-6.1595, -2.3495)
  line L7 (-6.1595, -2.3495) -> (-6.1595, 0)
  circle A0 centre (-13.335, -6.35) radius 2.05
  line L8 (-3.7465, -10.3505) -> (-22.9235, -10.3505)
  line L9 (-22.9235, -10.3505) -> (-22.9235, -9.8425)
  line L10 (-22.9235, -9.8425) -> (-3.7465, -9.8425)
  line L11 (-3.7465, -9.8425) -> (-3.7465, -10.3505)
  dimension "d82" = 0.508
  constraint horizontal L8
  constraint vertical L9
  constraint horizontal L10
  constraint vertical L11
  constraint coincident L4.end L5.start
  measures "d82" distance of L4.end L10.end
extrude "Extrude20" cut sketch "Sketch13" against normal up to surface (19.558 mm away) contours L3 L4 L5 L8 L9 L10 L11
extrude "Extrude21" add 1 faces at (26.8817, 9.525, -7.62) along direction (0, 0, -1) up to surface (1.27 mm away)
